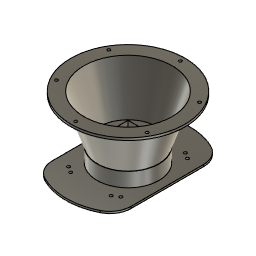
Cone Bottom (Autodesk Fusion 360 design; units mm, degrees)
Autodesk Fusion 360 part; units mm, degrees
note: some values were not read from the file. Chosen so that the rebuilt part matches the saved one: which face or edge a step refers to. Set by a fixed rule: which sketch regions a step uses.
sketch "Sketch1" plane through (0, 0, 0) normal (0, 1, 0) x (1, 0, 0)
  line L0 (0, 0) -> (32.2, 0)
  line L1 (0, 0) -> (0, -50)
  line L2 (48.95, -50) -> (32.2, 0)
  line L3 (0, -50) -> (48.95, -50)
  dimension "d1" = 32.2
  dimension "d142" = 50
  dimension "d143" = 48.95
  constraint coincident L0.start L1.start
  constraint horizontal L0
  constraint perpendicular L0 L1
  measures "d1" distance of L0.start L0.end
  measures "d142" distance of L0.start L1.end
  measures "d143" distance of L1.end L2.start
revolve "Revolve1" add sketch "Sketch1" angle 360 about axis through (0, 0, 0) along (0, 0, 1) makes body 1
shell "Shell1" thickness 2.5 removed faces 1 at (25.1837, 4.0906, 50) on bodies 1
sketch "Sketch2" plane through (0, 0, 0) normal (0, 0, -1) x (1, 0, 0)
  circle A0 centre (0, 0) radius 32.2
  line L0 (-21, -21) -> (21, -21)
  line L1 (21, -21) -> (21, 21)
  line L2 (21, 21) -> (-21, 21)
  line L3 (-21, 21) -> (-21, -21)
  circle A1 centre (0, 0) radius 32.5
  dimension "d6" = 42
  dimension "d7" = 42
  constraint horizontal L0
  constraint vertical L1
  constraint horizontal L2
  constraint vertical L3
  constraint coincident A0.centre A1.centre
  measures "d6" distance of L0.start L0.end
  measures "d7" distance of L0.start L2.end
extrude "Extrude1" add sketch "Sketch2" along normal blind 22.5 contours A0 | L0 L1 L2 L3 | A1 bodies 1
extrude "Extrude2" cut sketch "Sketch2" against normal blind 10 contours L0 L1 L2 L3 bodies 1
extrude "Extrude3" cut sketch "Sketch2" along normal blind 16 contours L0 L1 L2 L3 bodies 1
sketch "Sketch5" plane through (0, 0, -16) normal (0, 0, 1) x (-1, 0, 0)
  line L0 (21, -21) -> (21, 21)
  line L1 (21, 21) -> (-21, 21)
  line L2 (-21, 21) -> (-21, -21)
  line L3 (-21, -21) -> (21, -21)
  circle A0 centre (17.5, -17.5) radius 1.5
  circle A1 centre (-17.5, -17.5) radius 1.5
  circle A2 centre (17.5, 17.5) radius 1.5
  circle A3 centre (-17.5, 17.5) radius 1.5
  line L4 (21, 21) -> (28.894, 21) construction
  line L5 (18.4952, 13.5139) -> (3.4952, 13.5139)
  line L6 (3.4952, 13.5139) -> (3.4952, -1.4861)
  line L7 (3.4952, -1.4861) -> (18.4952, -1.4861)
  line L8 (18.4952, -1.4861) -> (18.4952, 13.5139)
  dimension "d17" = 15
  dimension "d18" = 15
  constraint horizontal L4
  constraint coincident L0.end L1.start
  constraint horizontal L5
  constraint vertical L6
  constraint horizontal L7
  constraint vertical L8
  measures "d17" distance of L5.start L5.end
  measures "d18" distance of L5.start L7.end
extrude "Extrude4" cut sketch "Sketch5" against normal blind 1 contours A0 | A1 | A2 | A3 | L5 L6 L7 L8 bodies 1
extrude "Extrude5" cut 1 faces at (-1.1612, -8.4698, -22.5) along direction (0, 0, 1) blind 5.5 on bodies 1 bodies 1
sketch "Sketch6" plane through (0, 0, -17) normal (0, 0, -1) x (1, 0, 0)
  circle A0 centre (-17.5, -17.5) radius 1.5
  line L0 (-18.4952, 13.5139) -> (-3.4952, 13.5139)
  line L1 (-3.4952, 13.5139) -> (-3.4952, -1.4861)
  line L2 (-3.4952, -1.4861) -> (-18.4952, -1.4861)
  line L3 (-18.4952, -1.4861) -> (-18.4952, 13.5139)
  circle A1 centre (17.5, -17.5) radius 1.5
  circle A2 centre (-17.5, 17.5) radius 1.5
  circle A3 centre (17.5, 17.5) radius 1.5
  circle A4 centre (0, 0) radius 32.5
  line L4 (-18.4952, 13.5139) -> (-3.4952, 13.5139)
  line L5 (-3.4952, 13.5139) -> (-3.4952, -1.4861)
  line L6 (-3.4952, -1.4861) -> (-18.4952, -1.4861)
  line L7 (-18.4952, -1.4861) -> (-18.4952, 13.5139)
  circle A5 centre (-17.5, 17.5) radius 1.5
  circle A6 centre (17.5, 17.5) radius 1.5
  circle A7 centre (17.5, -17.5) radius 1.5
  circle A8 centre (-17.5, -17.5) radius 1.5
  circle A9 centre (0, 0) radius 65
  line L8 (0, 0) -> (44.414, 0) construction
  line L9 (0, 0) -> (44.414, 0) construction
  line L10 (0, 0) -> (44.414, 0) construction
  line L11 (0, 0) -> (44.414, 0) construction
  circle A10 centre (21.2606, -38.9947) radius 1.5
  circle A11 centre (-21.2606, -38.9947) radius 1.5
  circle A12 centre (-21.2606, 38.9947) radius 1.5
  circle A13 centre (21.2606, 38.9947) radius 1.5
  line L12 (0, 0) -> (65, 0)
  line L13 (0, 0) -> (0, 65)
  line L14 (0, -65) -> (0, 0)
  line L15 (0, 0) -> (-65, 0)
  dimension "d23" = 130
  dimension "d32" = 3
  dimension "d33" = 3
  dimension "d34" = 3
  dimension "d35" = 3
  constraint horizontal L4
  constraint vertical L5
  constraint horizontal L6
  constraint vertical L7
  constraint coincident L1.end L2.start
  constraint coincident L0.start L3.end
  constraint concentric A2 A5
  constraint concentric A3 A6
  constraint concentric A1 A7
  constraint concentric A0 A8
  constraint coincident A4.centre A9.centre
  constraint horizontal L8
  constraint horizontal L9
  constraint horizontal L10
  constraint horizontal L11
  constraint coincident A9 L12.end
  constraint parallel L9 L12
  constraint coincident A9 L13.end
  constraint perpendicular L10 L13
  constraint coincident A9 L14.start
  constraint perpendicular L12 L14
  constraint coincident A9 L15.end
  constraint perpendicular L5 L15
  measures "d23" diameter of A9
  measures "d32" diameter of A10
  measures "d33" diameter of A11
  measures "d34" diameter of A12
  measures "d35" diameter of A13
extrude "Extrude6" add sketch "Sketch6" against normal blind 2 contours A4 A9 L13 L15 | A4 A9 L14 L15 | A4 A9 L12 L13 | A4 A9 L12 L14 bodies 1
sketch "Sketch7" plane through (0, 0, -17) normal (0, 0, -1) x (1, 0, 0)
  circle A0 centre (0, 0) radius 65
  circle A1 centre (21.2606, 38.9947) radius 1.5
  circle A2 centre (-21.2606, 38.9947) radius 1.5
  circle A3 centre (21.2606, -38.9947) radius 1.5
  circle A4 centre (-21.2606, -38.9947) radius 1.5
  circle A5 centre (-17.5, -17.5) radius 1.5
  line L0 (-18.4952, 13.5139) -> (-3.4952, 13.5139)
  line L1 (-3.4952, 13.5139) -> (-3.4952, -1.4861)
  line L2 (-3.4952, -1.4861) -> (-18.4952, -1.4861)
  line L3 (-18.4952, -1.4861) -> (-18.4952, 13.5139)
  circle A6 centre (17.5, -17.5) radius 1.5
  circle A7 centre (-17.5, 17.5) radius 1.5
  circle A8 centre (17.5, 17.5) radius 1.5
  line L4 (0, 0) -> (41.407, 0)
  line L5 (0, 0) -> (-41.407, 0)
  line L6 (-41.407, 0) -> (-41.407, 50.1045)
  line L7 (-41.407, 0) -> (-41.407, -50.1045)
  line L8 (41.407, 0) -> (41.407, 50.1045)
  line L9 (41.407, 50.1045) -> (41.407, -50.1045)
  dimension "d38" = 41.407
  dimension "d39" = 41.407
  constraint coincident A0.centre L4.start
  constraint horizontal L4
  constraint parallel L4 L5
  constraint coincident A0 L6.end
  constraint perpendicular L5 L6
  constraint coincident A0 L7.end
  constraint perpendicular L5 L7
  constraint coincident A0 L8.end
  constraint perpendicular L4 L8
  constraint coincident A0 L9.end
  constraint perpendicular L4 L9
  measures "d38" distance of A0.centre L4.end
  measures "d39" distance of A0.centre L5.end
extrude "Extrude7" cut sketch "Sketch7" against normal blind 2 contours A0 L8 L9 | A0 L6 L7 bodies 1
fillet "Fillet1" radius 22.5 4 edges at (-41.407, -50.1045, -16) (41.407, -50.1045, -16) (41.407, 50.1045, -16) (-41.407, 50.1045, -16) on bodies 1
sketch "Sketch8" plane through (0, 0, 0) normal (0, 0, 1) x (1, 0, 0)
  circle A0 centre (0, -45) radius 8
extrude "Extrude18" add sketch "Sketch8" along normal blind 1 separate body makes body 2
sketch "Sketch17" plane through (0, 0, -17) normal (0, 0, -1) x (1, 0, 0)
  circle A0 centre (17.5, 17.5) radius 1.5
  circle A1 centre (-17.5, 17.5) radius 1.5
  circle A2 centre (17.5, -17.5) radius 1.5
  line L0 (-18.4952, 13.5139) -> (-3.4952, 13.5139)
  line L1 (-3.4952, 13.5139) -> (-3.4952, -1.4861)
  line L2 (-3.4952, -1.4861) -> (-18.4952, -1.4861)
  line L3 (-18.4952, -1.4861) -> (-18.4952, 13.5139)
  circle A3 centre (-17.5, -17.5) radius 1.5
  circle A4 centre (-21.2606, -38.9947) radius 1.5
  circle A5 centre (21.2606, -38.9947) radius 1.5
  circle A6 centre (-21.2606, 38.9947) radius 1.5
  circle A7 centre (21.2606, 38.9947) radius 1.5
  arc A8 (-41.407, -38.0628) -> (-28.9166, -58.2137) centre (-18.907, -38.0628) ccw
  arc A9 (-28.9166, -58.2137) -> (28.9166, -58.2137) centre (0, 0) ccw
  arc A10 (28.9166, -58.2137) -> (41.407, -38.0628) centre (18.907, -38.0628) ccw
  line L4 (41.407, -38.0628) -> (41.407, 38.0628)
  arc A11 (41.407, 38.0628) -> (28.9166, 58.2137) centre (18.907, 38.0628) ccw
  arc A12 (28.9166, 58.2137) -> (-28.9166, 58.2137) centre (0, 0) ccw
  arc A13 (-28.9166, 58.2137) -> (-41.407, 38.0628) centre (-18.907, 38.0628) ccw
  line L5 (-41.407, 38.0628) -> (-41.407, -38.0628)
  circle A14 centre (-27.5, 35) radius 1.5
  circle A15 centre (27.5, 35) radius 1.5
  circle A16 centre (-27.5, -35) radius 1.5
  circle A17 centre (27.5, -35) radius 1.5
  dimension "d92" = 55
  dimension "d93" = 70
  dimension "d94" = 3
  dimension "d95" = 3
  measures "d92" distance of A14.centre A15.centre
  measures "d93" distance of A15.centre A17.centre
  measures "d94" diameter of A16
  measures "d95" diameter of A17
extrude "Extrude20" cut sketch "Sketch17" against normal blind 2 contours A4 | A5 | A14 | A15 bodies 1
extrude "Extrude21" cut sketch "Sketch17" against normal blind 2 contours A16 | A17 bodies 1
ref_plane "WorkPlane3" through (0, 0, 47.5) normal (0, 0, 1) x (1, 0, 0)
sketch "Sketch30" plane through (0, 0, 47.5) normal (0, 0, 1) x (1, 0, 0)
  circle A0 centre (0, 0) radius 60
  circle A1 centre (0, 0) radius 46.7442
  dimension "d150" = 120
  constraint coincident A0.centre A1.centre
  constraint concentric A0 A1
  measures "d150" diameter of A0
extrude "Extrude32" add sketch "Sketch30" along normal blind 2.5 bodies 1
sketch "Sketch32" plane through (0, 0, 50) normal (0, 0, 1) x (-1, 0, 0)
  circle A0 centre (0, 0) radius 60
  circle A1 centre (0, 0) radius 46.3134
  circle A2 centre (0, 55) radius 1.5
  line L0 (0, 0) -> (0, 60)
  circle A3 centre (-47.6314, 27.5) radius 1.5
  circle A4 centre (-47.6314, -27.5) radius 1.5
  circle A5 centre (0, -55) radius 1.5
  circle A6 centre (47.6314, -27.5) radius 1.5
  circle A7 centre (47.6314, 27.5) radius 1.5
  dimension "d154" = 3
  dimension "d155" = 60
  dimension "d156" = 55
  dimension "d158" = 360
  constraint coincident A0.centre A1.centre
  constraint coincident A0 L0.end
  constraint vertical L0
  measures "d154" diameter of A2
  measures "d155" distance of A0.centre L0.end
  measures "d156" distance of A0.centre A2.centre
extrude "Extrude33" cut sketch "Sketch32" against normal up to surface (2.5 mm away) contours A2 L0 | A2 L0 | A3 | A4 | A5 | A6 | A7 bodies 1
hidden bodies 2
